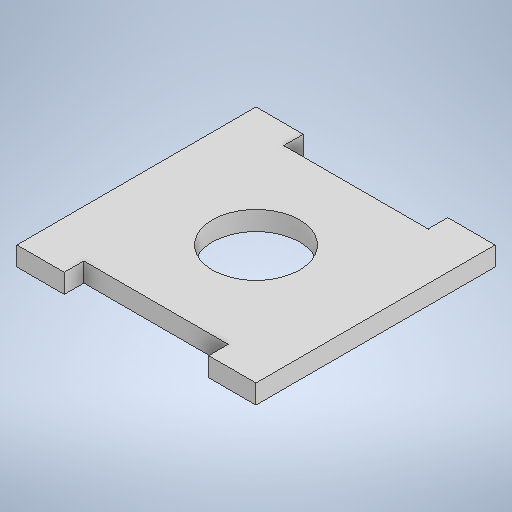
# Autodesk Inventor part: 센서 마운트
Saved by Autodesk Inventor 2025 (Build 290162000, 162)
## iProperties
Created: 2024-05-11
Part Number: 센서 마운트
Material: 일반
Document SubType Name: Modeling
Designer: gmsee
Density: 1 g/cm^3
Appearance: 기본값
Author: gmsee
Autodesk Inventor part; units mm, degrees
ref_plane "YZ Plane" through (0, 0, 0) normal (1, 0, 0) x (0, 1, 0)
ref_plane "XZ Plane" through (0, 0, 0) normal (0, 1, 0) x (-1, 0, 0)
ref_plane "XY Plane" through (0, 0, 0) normal (0, 0, 1) x (1, 0, 0)
sketch "스케치1" plane through (0, 0, 0) normal (0, 1, 0) x (-1, 0, 0)
  line L0 (25, 25) -> (-25, 25)
  line L1 (-25, 25) -> (-25, -25)
  line L2 (-25, -25) -> (25, -25)
  line L3 (25, -25) -> (25, 25)
  circle A0 centre (0, 0) radius 9.1
  line L4 (15.1, 25) -> (15.1, 20.9)
  line L5 (15.1, 20.9) -> (-15.1, 20.9)
  line L6 (-15.1, 20.9) -> (-15.1, 25)
  line L7 (15.1, -25) -> (15.1, -20.9)
  line L8 (15.1, -20.9) -> (-15.1, -20.9)
  line L9 (-15.1, -20.9) -> (-15.1, -25)
  point P0 (15.1, 22.95)
  point P1 (15.1, -22.95)
  dimension "d0" = 25
  dimension "d2" = 25
  dimension "d3" = 25
  dimension "d4" = 25
  dimension "d5" = 18.2
  dimension "d6" = 30.2
  dimension "d7" = 30.2
  dimension "d8" = 9.9
  dimension "d9" = 9.9
  dimension "d10" = 4.1
  dimension "d11" = 4.1
  constraints: 20 end point, 5 perpendicular, 4 point on line, 2 midpoint, 2 parallel, 2 vertical, 1 centre point, 1 coincident, 1 horizontal
  measures "d0" distance from line of L2 point (0, 0)
  measures "d2" distance from line of L0 point (0, 0)
  measures "d3" distance from line of L1 point (0, 0)
  measures "d4" distance from line of L3 point (0, 0)
  measures "d5" diameter of A0
  measures "d6" distance of L4.end L5.end
  measures "d7" distance of L7.end L8.end
  measures "d8" distance from line of L3 point (15.1, 22.95)
  measures "d9" distance from line of L3 point (15.1, -22.95)
  measures "d10" distance of L5.end L6.end
  measures "d11" distance of L8.end L9.end
extrude "돌출1" add sketch "스케치1" along normal blind 4 contours L3 L2 L7 L8 L9 L1 L0 L6 L5 L4
